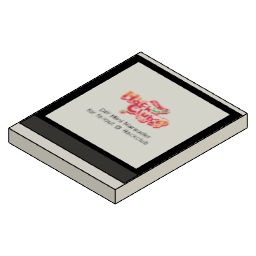
Showcase (Autodesk Fusion 360 archive; units mm, degrees)
design "Display"
Autodesk Fusion 360 part; units mm, degrees
sketch "Sketch1" plane through (0, 0, 0) normal (0, 0, 1) x (1, 0, 0)
  line L0 (14.765, 18.3) -> (-14.765, 18.3)
  line L1 (-14.765, 18.3) -> (-14.765, -18.3)
  line L2 (-14.765, -18.3) -> (14.765, -18.3)
  line L3 (14.765, -18.3) -> (14.765, 18.3)
  line L4 (14.765, 18.3) -> (-14.765, -18.3) construction
  line L5 (-14.765, 18.3) -> (14.765, -18.3) construction
  line L6 (12.765, 15.72) -> (-12.765, 15.72)
  line L7 (-12.765, -10.5) -> (12.765, -10.5)
  line L8 (12.765, -10.5) -> (12.765, 15.72)
  line L9 (-12.765, 15.72) -> (-12.765, -10.5)
  line L10 (14.445, -15.53) -> (14.445, 17.12)
  line L11 (-14.445, 17.12) -> (-14.445, -15.53)
  line L12 (14.445, 17.12) -> (-14.445, 17.12)
  line L13 (-14.445, -15.53) -> (14.445, -15.53)
  line L14 (-14.445, -11.53) -> (14.445, -11.53)
  dimension "d1" = 29.53
  dimension "d2" = 36.6
  dimension "d3" = -2.58
  dimension "d4" = -7.8
  dimension "d5" = -2
  dimension "d6" = -2
  dimension "d7" = -0.32
  dimension "d8" = -1.18
  dimension "d9" = -2.77
  dimension "d10" = -4
  constraint horizontal L0
  constraint perpendicular L0 L1
  constraint parallel L0 L2
  constraint parallel L1 L3
  constraint coincident L4 origin
  constraint coincident L5 origin
  constraint coincident L10.end L12
  constraint coincident L11.start L12
  constraint coincident L6 L9.start
  constraint coincident L6 L8.end
  constraint coincident L7 L8.start
  constraint coincident L7 L9.end
  constraint coincident L10 L13.end
  constraint coincident L11 L13.start
  measures "d1" distance of L1.end L2.end
  measures "d2" distance of L0.end L1.end
extrude "Extrude1" add sketch "Sketch1" along normal blind 3.47 contours L0 L1 L2 L3 makes body 1
extrude "Extrude2" add sketch "Sketch1" along normal blind 3.47 separate body contours L10 L11 L13 L14 makes body 2
extrude "Extrude3" add sketch "Sketch1" along normal blind 3.47 separate body contours L10 L11 L12 L14 makes body 3
extrude "Extrude4" add sketch "Sketch1" along normal blind 3.47 separate body contours L6 L7 L8 L9 makes body 4
named bodies: "Outer shell", "Ribbon Cover", "LEDs Frame", "LEDs"
